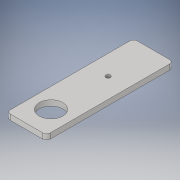
# Autodesk Inventor part: 12mero
Saved by Autodesk Inventor 2019 (Build 230136000, 136)
## iProperties
Created: 2022-09-04
Part Number: 12mero
Material: Generic
Document SubType Name: Modeling
Designer: laca
Density: 1 g/cm^3
Appearance: Default
Author: laca
Autodesk Inventor part; units mm, degrees
ref_plane "YZ Plane" through (0, 0, 0) normal (1, 0, 0) x (0, 1, 0)
ref_plane "XZ Plane" through (0, 0, 0) normal (0, 1, 0) x (-1, 0, 0)
ref_plane "XY Plane" through (0, 0, 0) normal (0, 0, 1) x (1, 0, 0)
sketch "Sketch1" plane through (0, 0, 0) normal (0, 1, 0) x (-1, 0, 0)
  line L0 (2, 0) -> (20, 0)
  line L1 (22, 2) -> (22, 68)
  line L2 (20, 70) -> (2, 70)
  line L3 (0, 68) -> (0, 2)
  circle A0 centre (11, 25) radius 1.25
  arc A1 (22, 68) -> (20, 70) centre (20, 68) ccw
  arc A2 (2, 70) -> (0, 68) centre (2, 68) ccw
  arc A3 (0, 2) -> (2, 0) centre (2, 2) ccw
  arc A4 (20, 0) -> (22, 2) centre (20, 2) ccw
  circle A5 centre (11, 56.5) radius 6.5
  point P0 (0, 0)
  point P1 (22, 70)
  point P2 (22, 0)
  dimension "d0" = 22
  dimension "d1" = 70
  dimension "d2" = 2.5
  dimension "d3" = 25
  dimension "d6" = 11
  dimension "d8" = 2
  dimension "d9" = 13
  dimension "d10" = 31.5
  constraints: 8 end point, 8 point on circle, 8 tangent, 6 centre point, 6 point on line, 3 equal radius, 2 parallel, 1 horizontal, 1 perpendicular
  measures "d0" distance between parallel lines of L3 L1
  measures "d1" distance of point (22, 0) point (22, 70)
  measures "d2" diameter of A0
  measures "d3" distance from line of L0 A0.centre
  measures "d6" distance from line of L3 A0.centre
  measures "d8" radius of A1
  measures "d9" diameter of A5
  measures "d10" distance of A0.centre A5.centre
extrude "Extrusion1" add sketch "Sketch1" along normal blind 3
equation "\"d6\" = 0.5 * d0"
body "Solid1"
